Autodesk Fusion 360 part; units mm, degrees
(part 3 of 14)
  arc A556 (6.35, 3.81) -> (6.35, 8.89) centre (6.35, 6.35) ccw
  arc A557 (6.35, 7.62) -> (6.35, 5.08) centre (6.35, 6.35) ccw
  line L1174 (33.239, 57.1172) -> (33.239, 57.7268)
  line L1175 (29.615, 19.102) -> (28.515, 19.102)
  line L1176 (33.872, 57.1172) -> (33.872, 57.7268)
  arc A558 (6.35, 5.08) -> (6.35, 7.62) centre (6.35, 6.35) ccw
  line L1177 (28.94, 19.5132) -> (29.19, 19.5132)
  arc A559 (6.35, 7.62) -> (6.35, 5.08) centre (6.35, 6.35) ccw
  line L1178 (29.615, 20.118) -> (28.515, 20.118)
  line L1179 (82.637, 29.083) -> (83.187, 29.083)
  line L1180 (29.615, 18.502) -> (29.615, 19.102)
  line L1181 (28.557, 18.4972) -> (28.557, 19.1068)
  line L1182 (29.573, 20.1228) -> (29.573, 19.5132)
  line L1183 (34.255, 57.7268) -> (34.255, 57.1172)
  line L1184 (29.573, 19.5132) -> (28.557, 19.5132)
  line L1185 (29.573, 19.1068) -> (29.573, 18.4972)
  line L1186 (83.437, 29.083) -> (83.987, 29.083)
  line L1187 (28.557, 20.1228) -> (29.573, 20.1228)
  arc A560 (34.2967, 57.722) -> (34.2972, 57.722) centre (34.297, 57.722) ccw
  arc A561 (33.1972, 57.122) -> (33.1967, 57.122) centre (33.197, 57.122) ccw
  arc A562 (8.6995, 11.684) -> (4.0005, 11.684) centre (6.35, 11.684) ccw
  line L1188 (33.239, 57.7268) -> (34.255, 57.7268)
  line L1189 (28.515, 18.502) -> (29.615, 18.502)
  line L1190 (28.557, 20.1228) -> (29.573, 20.1228)
  line L1191 (34.422, 57.422) -> (33.872, 57.422)
  line L1192 (29.19, 19.5132) -> (29.19, 20.1228)
  arc A563 (6.35, 6.6992) -> (6.35, 6.0007) centre (6.35, 6.35) ccw
  arc A564 (77.273, 25.0129) -> (77.273, 24.8351) centre (77.273, 24.924) ccw
  arc A565 (4.0005, 11.684) -> (8.6995, 11.684) centre (6.35, 11.684) ccw
  line L1193 (34.255, 57.7268) -> (34.255, 57.1172)
  line L1194 (28.94, 18.4972) -> (29.19, 18.4972)
  line L1195 (33.239, 57.7268) -> (34.255, 57.7268)
  line L1196 (34.255, 57.1172) -> (33.239, 57.1172)
  line L1197 (29.19, 18.4972) -> (29.19, 19.1068)
  line L1198 (28.515, 20.118) -> (28.515, 19.518)
  arc A566 (6.35, 8.89) -> (6.35, 3.81) centre (6.35, 6.35) ccw
  arc A567 (6.35, 5.08) -> (6.35, 7.62) centre (6.35, 6.35) ccw
  line L1199 (28.557, 20.5292) -> (28.557, 21.1388)
  line L1200 (33.872, 57.7268) -> (33.622, 57.7268)
  arc A568 (33.1967, 57.122) -> (33.1972, 57.122) centre (33.197, 57.122) ccw
  line L1201 (29.573, 19.1068) -> (29.573, 18.4972)
  line L1202 (82.637, 29.083) -> (83.187, 29.083)
  line L1203 (28.557, 19.5132) -> (28.557, 20.1228)
  arc A569 (33.1967, 57.722) -> (33.1972, 57.722) centre (33.197, 57.722) ccw
  arc A570 (77.273, 24.8351) -> (77.273, 25.0129) centre (77.273, 24.924) ccw
  line L1204 (29.573, 18.4972) -> (28.557, 18.4972)
  arc A571 (6.35, 3.81) -> (6.35, 8.89) centre (6.35, 6.35) ccw
  line L1205 (34.422, 57.422) -> (33.872, 57.422)
  line L1206 (33.622, 57.1172) -> (33.872, 57.1172)
  line L1207 (33.239, 57.1172) -> (33.239, 57.7268)
  line L1208 (34.255, 57.1172) -> (33.239, 57.1172)
  line L1209 (34.297, 57.722) -> (33.197, 57.722)
  line L1210 (33.197, 57.722) -> (33.197, 57.122)
  arc A572 (33.1972, 57.722) -> (33.1967, 57.722) centre (33.197, 57.722) ccw
  line L1211 (34.297, 57.122) -> (34.297, 57.722)
  line L1212 (28.94, 20.1228) -> (28.94, 19.5132)
  line L1213 (28.515, 19.102) -> (28.515, 18.502)
  arc A573 (6.35, 6.0007) -> (6.35, 6.6992) centre (6.35, 6.35) ccw
  line L1214 (29.615, 19.518) -> (29.615, 20.118)
  line L1215 (7.8317, 13.1657) -> (8.0113, 13.3453)
  line L1216 (28.557, 19.1068) -> (29.573, 19.1068)
  line L1217 (29.573, 20.5292) -> (28.557, 20.5292)
  line L1218 (29.573, 19.5132) -> (28.557, 19.5132)
  arc A574 (6.35, 8.89) -> (6.35, 3.81) centre (6.35, 6.35) ccw
  line L1219 (28.557, 19.5132) -> (28.557, 20.1228)
  arc A575 (6.35, 7.62) -> (6.35, 5.08) centre (6.35, 6.35) ccw
  line L1220 (29.19, 20.1228) -> (28.94, 20.1228)
  line L1221 (28.94, 19.1068) -> (28.94, 18.4972)
  arc A576 (6.35, 7.62) -> (6.35, 5.08) centre (6.35, 6.35) ccw
  line L1222 (29.573, 21.1388) -> (29.573, 20.5292)
  line L1223 (28.515, 21.134) -> (28.515, 20.534)
  arc A577 (78.9432, 34.3535) -> (78.9432, 34.4805) centre (78.9432, 34.417) ccw
  arc A578 (79.5528, 33.3375) -> (79.5528, 33.4645) centre (79.5528, 33.401) ccw
  arc A579 (79.5528, 34.4805) -> (79.5528, 34.3535) centre (79.5528, 34.417) ccw
  line L1224 (78.9432, 33.401) -> (78.9432, 34.417)
  arc A580 (79.5528, 33.4645) -> (79.5528, 33.3375) centre (79.5528, 33.401) ccw
  line L1225 (79.548, 33.359) -> (79.548, 34.459)
  line L1226 (79.5528, 33.401) -> (78.9432, 33.401)
  arc A581 (79.5528, 34.3535) -> (79.5528, 34.4805) centre (79.5528, 34.417) ccw
  line L1227 (79.548, 34.459) -> (78.948, 34.459)
  arc A582 (79.548, 33.3588) -> (79.548, 33.3592) centre (79.548, 33.359) ccw
  arc A583 (79.548, 33.3592) -> (79.548, 33.3588) centre (79.548, 33.359) ccw
  arc A584 (79.548, 34.4592) -> (79.548, 34.4588) centre (79.548, 34.459) ccw
  arc A585 (78.948, 34.4588) -> (78.948, 34.4592) centre (78.948, 34.459) ccw
  line L1228 (78.948, 34.459) -> (78.948, 33.359)
  arc A586 (78.948, 33.3588) -> (78.948, 33.3592) centre (78.948, 33.359) ccw
  arc A587 (79.548, 34.4588) -> (79.548, 34.4592) centre (79.548, 34.459) ccw
  line L1229 (78.948, 33.359) -> (79.548, 33.359)
  line L1230 (78.9432, 34.417) -> (79.5528, 34.417)
  arc A588 (78.9432, 34.4805) -> (78.9432, 34.3535) centre (78.9432, 34.417) ccw
  arc A589 (78.9432, 33.3375) -> (78.9432, 33.4645) centre (78.9432, 33.401) ccw
  arc A590 (78.9432, 33.4645) -> (78.9432, 33.3375) centre (78.9432, 33.401) ccw
  line L1231 (79.5528, 34.417) -> (79.5528, 33.401)
  arc A591 (94.5642, 21.0185) -> (94.5642, 20.8915) centre (94.5642, 20.955) ccw
  arc A592 (94.5642, 20.8915) -> (94.5642, 21.0185) centre (94.5642, 20.955) ccw
  line L1232 (94.5642, 20.572) -> (94.5642, 20.322)
  arc A593 (95.1738, 20.8915) -> (95.1738, 21.0185) centre (95.1738, 20.955) ccw
  line L1233 (94.5642, 20.322) -> (95.1738, 20.322)
  arc A594 (79.5528, 33.3375) -> (79.5528, 33.4645) centre (79.5528, 33.401) ccw
  line L1234 (0, 0) -> (101.6, 0)
  line L1235 (79.5528, 33.784) -> (79.5528, 34.034)
  line L1236 (95.1738, 20.572) -> (94.5642, 20.572)
  line L1237 (78.9432, 33.784) -> (79.5528, 33.784)
  arc A595 (95.1738, 21.0185) -> (95.1738, 20.8915) centre (95.1738, 20.955) ccw
  arc A596 (79.5528, 33.4645) -> (79.5528, 33.3375) centre (79.5528, 33.401) ccw
  line L1238 (0, 63.5) -> (0, 0)
  arc A597 (94.5642, 19.8755) -> (94.5642, 20.0025) centre (94.5642, 19.939) ccw
  line L1239 (101.6, 63.5) -> (0, 63.5)
  line L1240 (95.1738, 20.322) -> (95.1738, 20.572)
  line L1241 (101.6, 0) -> (101.6, 63.5)
  arc A598 (94.5642, 20.0025) -> (94.5642, 19.8755) centre (94.5642, 19.939) ccw
  arc A599 (-0.0635, 0) -> (0.0635, 0) centre (0, 0) ccw
  arc A600 (78.9432, 34.4805) -> (78.9432, 34.3535) centre (78.9432, 34.417) ccw
  arc A601 (78.948, 34.4592) -> (78.948, 34.4588) centre (78.948, 34.459) ccw
  line L1242 (94.869, 20.322) -> (94.869, 19.772)
  line L1243 (34.422, 57.422) -> (33.872, 57.422)
  arc A602 (78.9432, 34.3535) -> (78.9432, 34.4805) centre (78.9432, 34.417) ccw
  line L1244 (28.557, 20.5292) -> (28.557, 21.1388)
  line L1245 (94.869, 20.322) -> (94.869, 19.772)
  line L1246 (79.5528, 34.034) -> (78.9432, 34.034)
  arc A603 (95.1738, 19.8755) -> (95.1738, 20.0025) centre (95.1738, 19.939) ccw
  arc A604 (95.1738, 20.0025) -> (95.1738, 19.8755) centre (95.1738, 19.939) ccw
  arc A605 (78.948, 33.3592) -> (78.948, 33.3588) centre (78.948, 33.359) ccw
  line L1247 (72.39, 34.4805) -> (72.39, 38.481)
  line L1248 (70.612, 21.59) -> (70.612, 32.385)
  line L1249 (79.248, 33.234) -> (79.248, 33.784)
  line L1250 (20.193, 51.054) -> (25.527, 51.054)
  line L1251 (25.527, 49.149) -> (24.384, 49.149)
  line L1252 (7.874, 53.975) -> (7.874, 47.244)
  arc A606 (0.0635, 63.5) -> (-0.0635, 63.5) centre (0, 63.5) ccw
  line L1253 (70.993, 34.29) -> (71.1835, 34.4805)
  line L1254 (24.384, 49.149) -> (22.987, 47.752)
  line L1255 (71.1581, 19.5148) -> (70.9003, 19.7726)
  line L1256 (22.987, 47.752) -> (20.193, 47.752)
  line L1257 (70.9003, 19.7726) -> (68.3387, 19.7726)
  line L1258 (15.494, 35.814) -> (26.035, 35.814)
  line L1259 (86.3702, 32.9565) -> (86.3702, 36.957)
  line L1260 (82.2935, 36.957) -> (82.2935, 32.766)
  line L1261 (85.0265, 32.9565) -> (86.3702, 32.9565)
  line L1262 (82.169, 22.479) -> (84.963, 22.479)
  line L1263 (22.4155, 53.975) -> (7.874, 53.975)
  line L1264 (85.1535, 22.3012) -> (86.233, 22.3012)
  line L1265 (84.836, 32.766) -> (85.0265, 32.9565)
  line L1266 (71.1835, 34.4805) -> (72.39, 34.4805)
  line L1267 (81.407, 21.59) -> (70.612, 21.59)
  line L1268 (26.035, 35.814) -> (28.829, 37.592)
  line L1269 (20.193, 47.752) -> (20.193, 51.054)
  line L1270 (68.3387, 19.7726) -> (68.3387, 15.4991)
  line L1271 (25.527, 51.054) -> (25.527, 49.149)
  line L1272 (37.338, 45.974) -> (37.338, 41.656)
  line L1273 (37.338, 41.656) -> (39.6875, 39.3065)
  line L1274 (28.829, 37.592) -> (28.829, 43.18)
  line L1275 (9.017, 46.101) -> (20.193, 46.101)
  line L1276 (20.193, 46.101) -> (22.4155, 48.3235)
  arc A607 (101.5365, 0) -> (101.6635, 0) centre (101.6, 0) ccw
  arc A608 (101.5365, 63.5) -> (101.6635, 63.5) centre (101.6, 63.5) ccw
  arc A609 (-0.0635, 63.5) -> (0.0635, 63.5) centre (0, 63.5) ccw
  arc A610 (101.6635, 63.5) -> (101.5365, 63.5) centre (101.6, 63.5) ccw
  line L1277 (7.874, 47.244) -> (9.017, 46.101)
  line L1278 (13.335, 43.18) -> (13.335, 37.973)
  line L1279 (28.829, 43.18) -> (13.335, 43.18)
  line L1280 (22.4155, 48.3235) -> (22.4155, 53.975)
  arc A611 (101.6635, 0) -> (101.5365, 0) centre (101.6, 0) ccw
  line L1281 (13.335, 37.973) -> (15.494, 35.814)
  line L1282 (82.2935, 32.766) -> (84.836, 32.766)
  arc A612 (0.0635, 0) -> (-0.0635, 0) centre (0, 0) ccw
  line L1283 (86.3702, 36.957) -> (82.2935, 36.957)
  line L1284 (84.963, 22.479) -> (85.1535, 22.3012)
  line L1285 (86.233, 22.3012) -> (86.233, 18.415)
  line L1286 (86.233, 18.415) -> (82.169, 18.415)
  line L1287 (68.326, 34.29) -> (70.993, 34.29)
  line L1288 (72.39, 38.481) -> (68.326, 38.481)
  line L1289 (68.326, 38.481) -> (68.326, 34.29)
  line L1290 (68.3387, 15.4991) -> (72.3824, 15.4991)
  line L1291 (82.169, 18.415) -> (82.169, 22.479)
  arc A613 (95.169, 20.9968) -> (95.169, 20.9972) centre (95.169, 20.997) ccw
  line L1292 (94.5642, 20.955) -> (95.1738, 20.955)
  line L1293 (39.624, 43.053) -> (39.624, 45.974)
  line L1294 (65.1993, 50.5765) -> (67.752, 50.5765)
  arc A614 (78.9432, 33.3375) -> (78.9432, 33.4645) centre (78.9432, 33.401) ccw
  line L1295 (95.1738, 20.955) -> (95.1738, 19.939)
  line L1296 (78.9432, 34.417) -> (79.5528, 34.417)
  line L1297 (57.8307, 52.8345) -> (57.8307, 49.4081)
  arc A615 (95.169, 19.8968) -> (95.169, 19.8972) centre (95.169, 19.897) ccw
  arc A616 (94.569, 19.8968) -> (94.569, 19.8972) centre (94.569, 19.897) ccw
  arc A617 (95.1738, 19.8755) -> (95.1738, 20.0025) centre (95.1738, 19.939) ccw
  line L1298 (65.1993, 53.3552) -> (65.1993, 50.5765)
  line L1299 (94.869, 21.122) -> (94.869, 20.572)
  line L1300 (94.869, 21.122) -> (94.869, 20.572)
  line L1301 (94.869, 21.122) -> (94.869, 20.572)
  line L1302 (79.5528, 34.417) -> (79.5528, 33.401)
  arc A618 (16.3571, 17.0434) -> (17.054, 17.0434) centre (16.7056, 17.0434) ccw
  line L1303 (78.9432, 33.401) -> (78.9432, 34.417)
  line L1304 (94.869, 20.322) -> (94.869, 19.772)
  line L1305 (61.4655, 52.8345) -> (57.8307, 52.8345)
  line L1306 (95.169, 19.897) -> (95.169, 20.997)
  line L1307 (95.1738, 19.939) -> (94.5642, 19.939)
  line L1308 (94.569, 19.897) -> (95.169, 19.897)
  arc A619 (95.169, 19.8972) -> (95.169, 19.8968) centre (95.169, 19.897) ccw
  line L1309 (61.4655, 51.7639) -> (61.4655, 52.8345)
  line L1310 (41.275, 39.3065) -> (41.275, 41.402)
  line L1311 (60.5015, 51.7639) -> (61.4655, 51.7639)
  line L1312 (57.8307, 49.4081) -> (59.5782, 49.4081)
  arc A620 (95.169, 20.9972) -> (95.169, 20.9968) centre (95.169, 20.997) ccw
  arc A621 (20.798, 16.9748) -> (20.1011, 16.9748) centre (20.4495, 16.9748) ccw
  line L1313 (39.624, 45.974) -> (37.338, 45.974)
  line L1314 (59.5782, 49.4081) -> (59.5782, 50.8406)
  line L1315 (95.1738, 20.955) -> (95.1738, 19.939)
  arc A622 (95.1738, 20.0025) -> (95.1738, 19.8755) centre (95.1738, 19.939) ccw
  arc A623 (95.1738, 20.8915) -> (95.1738, 21.0185) centre (95.1738, 20.955) ccw
  line L1316 (79.5528, 33.401) -> (78.9432, 33.401)
  line L1317 (41.275, 41.402) -> (39.624, 43.053)
  arc A624 (94.569, 19.8972) -> (94.569, 19.8968) centre (94.569, 19.897) ccw
  line L1318 (39.6875, 39.3065) -> (41.275, 39.3065)
  arc A625 (20.1011, 16.9748) -> (20.798, 16.9748) centre (20.4495, 16.9748) ccw
  line L1319 (95.1738, 19.939) -> (94.5642, 19.939)
  line L1320 (94.569, 20.997) -> (94.569, 19.897)
  arc A626 (94.5642, 19.8755) -> (94.5642, 20.0025) centre (94.5642, 19.939) ccw
  arc A627 (78.9432, 33.4645) -> (78.9432, 33.3375) centre (78.9432, 33.401) ccw
  arc A628 (94.5642, 20.0025) -> (94.5642, 19.8755) centre (94.5642, 19.939) ccw
  line L1321 (59.5782, 50.8406) -> (60.5015, 51.7639)
  line L1322 (81.407, 32.385) -> (81.407, 21.59)
  arc A629 (94.5642, 21.0185) -> (94.5642, 20.8915) centre (94.5642, 20.955) ccw
  arc A630 (94.5642, 20.8915) -> (94.5642, 21.0185) centre (94.5642, 20.955) ccw
  line L1323 (67.752, 53.3552) -> (65.1993, 53.3552)
  arc A631 (17.054, 17.0434) -> (16.3571, 17.0434) centre (16.7056, 17.0434) ccw
  line L1324 (70.612, 32.385) -> (81.407, 32.385)
  arc A632 (94.569, 20.9968) -> (94.569, 20.9972) centre (94.569, 20.997) ccw
  line L1325 (67.752, 50.5765) -> (67.752, 53.3552)
  line L1326 (95.169, 20.997) -> (94.569, 20.997)
  line L1327 (94.5642, 20.955) -> (95.1738, 20.955)
  arc A633 (94.569, 20.9972) -> (94.569, 20.9968) centre (94.569, 20.997) ccw
  arc A634 (95.1738, 21.0185) -> (95.1738, 20.8915) centre (95.1738, 20.955) ccw
  line L1328 (94.5642, 19.939) -> (94.5642, 20.955)
  line L1329 (94.5642, 19.939) -> (94.5642, 20.955)
  line L1330 (93.98, 54.356) -> (95.758, 54.356)
  line L1331 (17.272, 13.081) -> (27.559, 13.081)
  line L1332 (93.853, 24.638) -> (93.853, 23.368)
  line L1333 (15.907, 41.0492) -> (15.907, 44.4528)
  line L1334 (14.129, 41.0492) -> (15.907, 41.0492)
  arc A635 (15.918, 41.0512) -> (15.918, 41.0507) centre (15.918, 41.051) ccw
  arc A636 (15.918, 44.4508) -> (15.918, 44.4513) centre (15.918, 44.451) ccw
  arc A637 (14.118, 44.4508) -> (14.118, 44.4513) centre (14.118, 44.451) ccw
  line L1335 (91.44, 54.61) -> (93.853, 54.61)
  line L1336 (79.248, 33.234) -> (79.248, 33.784)
  line L1337 (78.9432, 34.034) -> (78.9432, 33.784)
  arc A638 (15.907, 41.1127) -> (15.907, 40.9857) centre (15.907, 41.0492) ccw
  line L1338 (95.758, 51.816) -> (93.98, 51.816)
  line L1339 (91.44, 24.638) -> (93.853, 24.638)
  line L1340 (93.98, 21.844) -> (93.98, 24.384)
  line L1341 (95.758, 21.844) -> (93.98, 21.844)
  line L1342 (93.98, 40.894) -> (95.758, 40.894)
  line L1343 (91.313, 39.37) -> (93.726, 39.37)
  line L1344 (27.559, 23.241) -> (17.272, 23.241)
  line L1345 (62.103, 41.402) -> (62.103, 17.526)
  line L1346 (93.853, 53.34) -> (91.44, 53.34)
  line L1347 (93.726, 38.1) -> (91.313, 38.1)
  line L1348 (79.248, 33.234) -> (79.248, 33.784)
  line L1349 (62.103, 17.526) -> (38.354, 17.526)
  line L1350 (93.726, 39.37) -> (93.726, 38.1)
  line L1351 (38.354, 17.526) -> (38.354, 41.402)
  line L1352 (72.3824, 15.4991) -> (72.3824, 19.5148)
  line L1353 (94.107, 6.858) -> (94.107, 9.398)
  line L1354 (72.3824, 19.5148) -> (71.1581, 19.5148)
  line L1355 (93.98, 51.816) -> (93.98, 54.356)
  line L1356 (94.107, 9.525) -> (91.567, 9.525)
  arc A639 (79.5528, 34.3535) -> (79.5528, 34.4805) centre (79.5528, 34.417) ccw
  arc A640 (15.907, 44.3893) -> (15.907, 44.5163) centre (15.907, 44.4528) ccw
  line L1357 (91.44, 23.368) -> (91.44, 24.638)
  line L1358 (95.885, 9.398) -> (95.885, 6.858)
  line L1359 (93.98, 24.384) -> (95.758, 24.384)
  line L1360 (95.758, 24.384) -> (95.758, 21.844)
  line L1361 (93.98, 38.354) -> (93.98, 40.894)
  line L1362 (91.313, 38.1) -> (91.313, 39.37)
  line L1363 (95.758, 54.356) -> (95.758, 51.816)
  line L1364 (95.885, 6.858) -> (94.107, 6.858)
  line L1365 (17.272, 23.241) -> (17.272, 13.081)
  line L1366 (91.44, 53.34) -> (91.44, 54.61)
  line L1367 (27.559, 13.081) -> (27.559, 23.241)
  line L1368 (95.758, 40.894) -> (95.758, 38.354)
  line L1369 (38.354, 41.402) -> (62.103, 41.402)
  line L1370 (91.567, 10.795) -> (94.107, 10.795)
  line L1371 (93.853, 23.368) -> (91.44, 23.368)
  line L1372 (93.853, 54.61) -> (93.853, 53.34)
  line L1373 (94.107, 10.795) -> (94.107, 9.525)
  line L1374 (91.567, 9.525) -> (91.567, 10.795)
  arc A641 (79.5528, 34.4805) -> (79.5528, 34.3535) centre (79.5528, 34.417) ccw
  line L1375 (14.129, 41.0492) -> (15.907, 41.0492)
  arc A642 (14.129, 44.3893) -> (14.129, 44.5163) centre (14.129, 44.4528) ccw
  line L1376 (14.129, 44.4528) -> (14.129, 41.0492)
  line L1377 (15.918, 41.051) -> (15.918, 44.451)
  line L1378 (14.129, 44.4528) -> (14.129, 41.0492)
  line L1379 (15.907, 44.4528) -> (14.129, 44.4528)
  line L1380 (95.758, 38.354) -> (93.98, 38.354)
  line L1381 (94.107, 9.398) -> (95.885, 9.398)
  arc A643 (23.992, 42.9753) -> (23.992, 42.9748) centre (23.992, 42.975) ccw
  arc A644 (14.129, 44.5163) -> (14.129, 44.3893) centre (14.129, 44.4528) ccw
  arc A645 (14.118, 44.4513) -> (14.118, 44.4508) centre (14.118, 44.451) ccw
  arc A646 (14.129, 40.9857) -> (14.129, 41.1127) centre (14.129, 41.0492) ccw
  line L1382 (14.168, 41.351) -> (15.868, 41.351)
  arc A647 (25.792, 42.9753) -> (25.792, 42.9748) centre (25.792, 42.975) ccw
  line L1383 (15.918, 44.451) -> (14.118, 44.451)
  arc A648 (15.907, 40.9857) -> (15.907, 41.1127) centre (15.907, 41.0492) ccw
  line L1384 (14.118, 41.051) -> (15.918, 41.051)
  arc A649 (25.792, 39.5752) -> (25.792, 39.5747) centre (25.792, 39.575) ccw
  line L1385 (23.992, 42.975) -> (23.992, 39.575)
  arc A650 (15.907, 41.1127) -> (15.907, 40.9857) centre (15.907, 41.0492) ccw
  line L1386 (14.168, 44.151) -> (15.868, 44.151)
  line L1387 (24.003, 39.5732) -> (25.781, 39.5732)
  line L1388 (25.781, 39.5732) -> (25.781, 42.9768)
  arc A651 (23.992, 39.5747) -> (23.992, 39.5752) centre (23.992, 39.575) ccw
  line L1389 (25.781, 42.9768) -> (24.003, 42.9768)
  arc A652 (25.792, 42.9748) -> (25.792, 42.9753) centre (25.792, 42.975) ccw
  arc A653 (24.003, 39.5097) -> (24.003, 39.6367) centre (24.003, 39.5732) ccw
  arc A654 (25.781, 39.6367) -> (25.781, 39.5097) centre (25.781, 39.5732) ccw
  arc A655 (24.003, 39.6367) -> (24.003, 39.5097) centre (24.003, 39.5732) ccw
  arc A656 (25.781, 43.0403) -> (25.781, 42.9133) centre (25.781, 42.9768) ccw
  arc A657 (24.003, 42.9133) -> (24.003, 43.0403) centre (24.003, 42.9768) ccw
  arc A658 (24.003, 43.0403) -> (24.003, 42.9133) centre (24.003, 42.9768) ccw
  arc A659 (14.129, 44.5163) -> (14.129, 44.3893) centre (14.129, 44.4528) ccw
  arc A660 (25.792, 39.5747) -> (25.792, 39.5752) centre (25.792, 39.575) ccw
  arc A661 (23.992, 42.9748) -> (23.992, 42.9753) centre (23.992, 42.975) ccw
  line L1390 (24.003, 42.9768) -> (24.003, 39.5732)
  arc A662 (14.129, 41.1127) -> (14.129, 40.9857) centre (14.129, 41.0492) ccw
  arc A663 (14.129, 44.3893) -> (14.129, 44.5163) centre (14.129, 44.4528) ccw
  arc A664 (15.907, 44.3893) -> (15.907, 44.5163) centre (15.907, 44.4528) ccw
  arc A665 (14.129, 44.5163) -> (14.129, 44.3893) centre (14.129, 44.4528) ccw
  arc A666 (14.129, 44.5163) -> (14.129, 44.3893) centre (14.129, 44.4528) ccw
  line L1391 (14.168, 41.351) -> (15.868, 41.351)
  line L1392 (14.118, 44.451) -> (14.118, 41.051)
  arc A667 (15.918, 41.0507) -> (15.918, 41.0512) centre (15.918, 41.051) ccw
  arc A668 (15.907, 44.5163) -> (15.907, 44.3893) centre (15.907, 44.4528) ccw
  arc A669 (14.118, 41.0507) -> (14.118, 41.0512) centre (14.118, 41.051) ccw
  arc A670 (14.129, 41.1127) -> (14.129, 40.9857) centre (14.129, 41.0492) ccw
  line L1393 (25.792, 39.575) -> (25.792, 42.975)
  line L1394 (14.168, 44.151) -> (15.868, 44.151)
  arc A671 (14.129, 44.3893) -> (14.129, 44.5163) centre (14.129, 44.4528) ccw
  arc A672 (23.992, 39.5752) -> (23.992, 39.5747) centre (23.992, 39.575) ccw
  line L1395 (15.907, 41.0492) -> (15.907, 44.4528)
  line L1396 (15.907, 44.4528) -> (14.129, 44.4528)
  arc A673 (15.907, 44.5163) -> (15.907, 44.3893) centre (15.907, 44.4528) ccw
  arc A674 (14.129, 44.3893) -> (14.129, 44.5163) centre (14.129, 44.4528) ccw
  line L1397 (79.248, 34.034) -> (79.248, 34.584)
  arc A675 (15.918, 44.4513) -> (15.918, 44.4508) centre (15.918, 44.451) ccw
  arc A676 (14.129, 40.9857) -> (14.129, 41.1127) centre (14.129, 41.0492) ccw
  line L1398 (79.248, 34.034) -> (79.248, 34.584)
  arc A677 (14.118, 41.0512) -> (14.118, 41.0507) centre (14.118, 41.051) ccw
  arc A678 (15.907, 40.9857) -> (15.907, 41.1127) centre (15.907, 41.0492) ccw
  line L1399 (79.248, 34.034) -> (79.248, 34.584)
  line L1400 (14.168, 44.151) -> (15.868, 44.151)
  line L1401 (23.992, 39.575) -> (25.792, 39.575)
  line L1402 (25.792, 42.975) -> (23.992, 42.975)
  line L1403 (14.168, 41.351) -> (15.868, 41.351)
  line L1404 (24.042, 42.675) -> (25.742, 42.675)
  arc A679 (10.922, 53.4543) -> (10.922, 53.5813) centre (10.922, 53.5178) ccw
  line L1405 (9.144, 53.5178) -> (9.144, 50.1142)
  line L1406 (9.133, 50.116) -> (10.933, 50.116)
  arc A680 (9.144, 53.5813) -> (9.144, 53.4543) centre (9.144, 53.5178) ccw
  line L1407 (24.042, 39.875) -> (25.742, 39.875)
  arc A681 (9.144, 50.1777) -> (9.144, 50.0507) centre (9.144, 50.1142) ccw
  arc A682 (24.003, 43.0403) -> (24.003, 42.9133) centre (24.003, 42.9768) ccw
  arc A683 (9.144, 53.4543) -> (9.144, 53.5813) centre (9.144, 53.5178) ccw
  line L1408 (24.003, 42.9768) -> (24.003, 39.5732)
  line L1409 (25.781, 42.9768) -> (24.003, 42.9768)
  line L1410 (10.922, 50.1142) -> (10.922, 53.5178)
  arc A684 (10.922, 53.4543) -> (10.922, 53.5813) centre (10.922, 53.5178) ccw
  arc A685 (10.922, 50.0507) -> (10.922, 50.1777) centre (10.922, 50.1142) ccw
  arc A686 (10.933, 50.1157) -> (10.933, 50.1162) centre (10.933, 50.116) ccw
  line L1411 (9.133, 53.516) -> (9.133, 50.116)
  arc A687 (9.133, 53.5163) -> (9.133, 53.5158) centre (9.133, 53.516) ccw
  arc A688 (9.133, 53.5158) -> (9.133, 53.5163) centre (9.133, 53.516) ccw
  arc A689 (24.003, 42.9133) -> (24.003, 43.0403) centre (24.003, 42.9768) ccw
  arc A690 (25.781, 39.5097) -> (25.781, 39.6367) centre (25.781, 39.5732) ccw
  arc A691 (9.144, 53.5813) -> (9.144, 53.4543) centre (9.144, 53.5178) ccw
  arc A692 (24.003, 42.9133) -> (24.003, 43.0403) centre (24.003, 42.9768) ccw
  arc A693 (24.003, 43.0403) -> (24.003, 42.9133) centre (24.003, 42.9768) ccw
  arc A694 (10.933, 50.1162) -> (10.933, 50.1157) centre (10.933, 50.116) ccw
  arc A695 (9.144, 53.4543) -> (9.144, 53.5813) centre (9.144, 53.5178) ccw
  arc A696 (9.144, 50.1777) -> (9.144, 50.0507) centre (9.144, 50.1142) ccw
  line L1412 (10.922, 53.5178) -> (9.144, 53.5178)
  arc A697 (9.144, 50.0507) -> (9.144, 50.1777) centre (9.144, 50.1142) ccw
  line L1413 (24.042, 42.675) -> (25.742, 42.675)
  arc A698 (10.922, 50.1777) -> (10.922, 50.0507) centre (10.922, 50.1142) ccw
  arc A699 (9.144, 53.5813) -> (9.144, 53.4543) centre (9.144, 53.5178) ccw
  arc A700 (24.003, 43.0403) -> (24.003, 42.9133) centre (24.003, 42.9768) ccw
  line L1414 (10.933, 50.116) -> (10.933, 53.516)
  arc A701 (10.922, 50.0507) -> (10.922, 50.1777) centre (10.922, 50.1142) ccw
  arc A702 (10.922, 53.5813) -> (10.922, 53.4543) centre (10.922, 53.5178) ccw
  arc A703 (10.933, 53.5163) -> (10.933, 53.5158) centre (10.933, 53.516) ccw
  arc A704 (10.922, 50.1777) -> (10.922, 50.0507) centre (10.922, 50.1142) ccw
  line L1415 (24.003, 39.5732) -> (25.781, 39.5732)
  arc A705 (10.933, 53.5158) -> (10.933, 53.5163) centre (10.933, 53.516) ccw
  arc A706 (9.133, 50.1162) -> (9.133, 50.1157) centre (9.133, 50.116) ccw
  arc A707 (9.144, 53.4543) -> (9.144, 53.5813) centre (9.144, 53.5178) ccw
  arc A708 (25.781, 42.9133) -> (25.781, 43.0403) centre (25.781, 42.9768) ccw
  arc A709 (25.781, 39.6367) -> (25.781, 39.5097) centre (25.781, 39.5732) ccw
  arc A710 (24.003, 39.6367) -> (24.003, 39.5097) centre (24.003, 39.5732) ccw
  line L1416 (25.781, 39.5732) -> (25.781, 42.9768)
  line L1417 (24.042, 39.875) -> (25.742, 39.875)
  line L1418 (9.144, 50.1142) -> (10.922, 50.1142)
  line L1419 (9.144, 53.5178) -> (9.144, 50.1142)
  arc A711 (25.781, 39.5097) -> (25.781, 39.6367) centre (25.781, 39.5732) ccw
  arc A712 (9.144, 50.0507) -> (9.144, 50.1777) centre (9.144, 50.1142) ccw
  line L1420 (24.042, 42.675) -> (25.742, 42.675)
  arc A713 (24.003, 39.5097) -> (24.003, 39.6367) centre (24.003, 39.5732) ccw
  arc A714 (24.003, 42.9133) -> (24.003, 43.0403) centre (24.003, 42.9768) ccw
  line L1421 (10.933, 53.516) -> (9.133, 53.516)
  arc A715 (25.781, 43.0403) -> (25.781, 42.9133) centre (25.781, 42.9768) ccw
  line L1422 (10.922, 53.5178) -> (9.144, 53.5178)
  arc A716 (25.781, 42.9133) -> (25.781, 43.0403) centre (25.781, 42.9768) ccw
  line L1423 (24.042, 39.875) -> (25.742, 39.875)
  line L1424 (80.564, 33.359) -> (80.564, 34.459)
  arc A717 (79.964, 34.4592) -> (79.964, 34.4588) centre (79.964, 34.459) ccw
  line L1425 (79.9592, 34.417) -> (80.5688, 34.417)
  line L1426 (79.9592, 33.401) -> (79.9592, 34.417)
  line L1427 (80.5688, 34.417) -> (80.5688, 33.401)
  line L1428 (80.264, 34.034) -> (80.264, 34.584)
  arc A718 (80.5688, 34.3535) -> (80.5688, 34.4805) centre (80.5688, 34.417) ccw
  line L1429 (20.18, 51.238) -> (21.98, 51.238)
  line L1430 (79.9592, 33.401) -> (79.9592, 34.417)
  line L1431 (80.264, 33.234) -> (80.264, 33.784)
  line L1432 (10.922, 50.1142) -> (10.922, 53.5178)
  arc A719 (79.9592, 33.4645) -> (79.9592, 33.3375) centre (79.9592, 33.401) ccw
  arc A720 (9.144, 53.5813) -> (9.144, 53.4543) centre (9.144, 53.5178) ccw
  arc A721 (79.964, 34.4588) -> (79.964, 34.4592) centre (79.964, 34.459) ccw
  line L1433 (80.264, 33.234) -> (80.264, 33.784)
  line L1434 (9.183, 50.416) -> (10.883, 50.416)
  line L1435 (80.5688, 33.401) -> (79.9592, 33.401)
  arc A722 (79.9592, 33.4645) -> (79.9592, 33.3375) centre (79.9592, 33.401) ccw
  line L1436 (20.18, 54.638) -> (20.18, 51.238)
  line L1437 (79.9592, 34.417) -> (80.5688, 34.417)
  line L1438 (9.183, 50.416) -> (10.883, 50.416)
  line L1439 (80.5688, 33.784) -> (80.5688, 34.034)
  arc A723 (79.9592, 34.4805) -> (79.9592, 34.3535) centre (79.9592, 34.417) ccw
  arc A724 (79.9592, 33.3375) -> (79.9592, 33.4645) centre (79.9592, 33.401) ccw
  arc A725 (80.564, 34.4588) -> (80.564, 34.4592) centre (80.564, 34.459) ccw
  arc A726 (79.9592, 34.3535) -> (79.9592, 34.4805) centre (79.9592, 34.417) ccw
  arc A727 (80.5688, 33.3375) -> (80.5688, 33.4645) centre (80.5688, 33.401) ccw
  line L1440 (80.264, 34.034) -> (80.264, 34.584)
  arc A728 (10.922, 53.5813) -> (10.922, 53.4543) centre (10.922, 53.5178) ccw
  line L1441 (9.183, 53.216) -> (10.883, 53.216)
  line L1442 (80.5688, 34.417) -> (80.5688, 33.401)
  arc A729 (9.133, 50.1157) -> (9.133, 50.1162) centre (9.133, 50.116) ccw
  line L1443 (80.5688, 33.401) -> (79.9592, 33.401)
  arc A730 (9.144, 53.4543) -> (9.144, 53.5813) centre (9.144, 53.5178) ccw
  arc A731 (79.964, 33.3588) -> (79.964, 33.3592) centre (79.964, 33.359) ccw
  arc A732 (80.5688, 33.4645) -> (80.5688, 33.3375) centre (80.5688, 33.401) ccw
  arc A733 (80.5688, 33.3375) -> (80.5688, 33.4645) centre (80.5688, 33.401) ccw
  arc A734 (79.964, 33.3592) -> (79.964, 33.3588) centre (79.964, 33.359) ccw
  arc A735 (79.9592, 33.3375) -> (79.9592, 33.4645) centre (79.9592, 33.401) ccw
  arc A736 (79.9592, 34.3535) -> (79.9592, 34.4805) centre (79.9592, 34.417) ccw
  line L1444 (9.144, 50.1142) -> (10.922, 50.1142)
  line L1445 (80.564, 34.459) -> (79.964, 34.459)
  line L1446 (79.9592, 33.784) -> (80.5688, 33.784)
  line L1447 (79.964, 33.359) -> (80.564, 33.359)
  arc A737 (80.5688, 33.4645) -> (80.5688, 33.3375) centre (80.5688, 33.401) ccw
  line L1448 (9.183, 50.416) -> (10.883, 50.416)
  line L1449 (9.183, 53.216) -> (10.883, 53.216)
  arc A738 (80.5688, 34.4805) -> (80.5688, 34.3535) centre (80.5688, 34.417) ccw
  line L1450 (80.5688, 34.034) -> (79.9592, 34.034)
  line L1451 (79.964, 34.459) -> (79.964, 33.359)
  arc A739 (80.564, 33.3588) -> (80.564, 33.3592) centre (80.564, 33.359) ccw
  arc A740 (80.564, 33.3592) -> (80.564, 33.3588) centre (80.564, 33.359) ccw
  line L1452 (9.183, 53.216) -> (10.883, 53.216)
  arc A741 (80.564, 34.4592) -> (80.564, 34.4588) centre (80.564, 34.459) ccw
  arc A742 (79.9592, 34.4805) -> (79.9592, 34.3535) centre (79.9592, 34.417) ccw
  line L1453 (80.264, 33.234) -> (80.264, 33.784)
  line L1454 (80.264, 34.034) -> (80.264, 34.584)
  arc A743 (80.5688, 34.4805) -> (80.5688, 34.3535) centre (80.5688, 34.417) ccw
  line L1455 (79.9592, 34.034) -> (79.9592, 33.784)
  arc A744 (80.5688, 34.3535) -> (80.5688, 34.4805) centre (80.5688, 34.417) ccw
  arc A745 (21.969, 51.2997) -> (21.969, 51.1727) centre (21.969, 51.2362) ccw
  arc A746 (3.048, 52.3875) -> (3.048, 52.5145) centre (3.048, 52.451) ccw
  line L1456 (21.969, 54.6398) -> (20.191, 54.6398)
  line L1457 (3.048, 44.831) -> (7.62, 44.831)
  line L1458 (3.048, 52.451) -> (3.048, 44.831)
  arc A747 (3.048, 52.5145) -> (3.048, 52.3875) centre (3.048, 52.451) ccw
  arc A748 (3.048, 52.3875) -> (3.048, 52.5145) centre (3.048, 52.451) ccw
  arc A749 (20.191, 54.5763) -> (20.191, 54.7033) centre (20.191, 54.6398) ccw
  line L1459 (7.5946, 51.8668) -> (7.5946, 52.0446)
  line L1460 (21.969, 54.6398) -> (20.191, 54.6398)
  line L1461 (20.23, 54.338) -> (21.93, 54.338)
  line L1462 (20.191, 51.2362) -> (21.969, 51.2362)
  line L1463 (3.1242, 52.0446) -> (3.1242, 52.2478)
  line L1464 (20.23, 54.338) -> (21.93, 54.338)
  arc A750 (7.5946, 51.9303) -> (7.5946, 51.8033) centre (7.5946, 51.8668) ccw
  arc A751 (3.048, 44.8945) -> (3.048, 44.7675) centre (3.048, 44.831) ccw
  line L1465 (7.62, 44.831) -> (7.62, 52.451)
  arc A752 (3.1242, 52.1081) -> (3.1242, 51.9811) centre (3.1242, 52.0446) ccw
  arc A753 (7.5946, 52.1081) -> (7.5946, 51.9811) centre (7.5946, 52.0446) ccw
  arc A754 (20.191, 54.5763) -> (20.191, 54.7033) centre (20.191, 54.6398) ccw
  arc A755 (20.191, 54.7033) -> (20.191, 54.5763) centre (20.191, 54.6398) ccw
  arc A756 (21.969, 51.2997) -> (21.969, 51.1727) centre (21.969, 51.2362) ccw
  arc A757 (20.191, 51.2997) -> (20.191, 51.1727) centre (20.191, 51.2362) ccw
  line L1466 (21.98, 51.238) -> (21.98, 54.638)
  arc A758 (20.191, 51.1727) -> (20.191, 51.2997) centre (20.191, 51.2362) ccw
  line L1467 (20.191, 54.6398) -> (20.191, 51.2362)
  line L1468 (3.0988, 51.8668) -> (7.5946, 51.8668)
  line L1469 (21.969, 51.2362) -> (21.969, 54.6398)
  line L1470 (20.191, 54.6398) -> (20.191, 51.2362)
  arc A759 (20.191, 54.7033) -> (20.191, 54.5763) centre (20.191, 54.6398) ccw
  line L1471 (20.23, 54.338) -> (21.93, 54.338)
  line L1472 (3.1242, 52.2478) -> (7.5946, 52.2478)
  arc A760 (21.969, 54.5763) -> (21.969, 54.7033) centre (21.969, 54.6398) ccw
  arc A761 (3.1242, 52.3113) -> (3.1242, 52.1843) centre (3.1242, 52.2478) ccw
  arc A762 (3.048, 52.5145) -> (3.048, 52.3875) centre (3.048, 52.451) ccw
  arc A763 (7.62, 44.8945) -> (7.62, 44.7675) centre (7.62, 44.831) ccw
  line L1473 (20.23, 51.538) -> (21.93, 51.538)
  arc A764 (21.969, 51.1727) -> (21.969, 51.2997) centre (21.969, 51.2362) ccw
  arc A765 (21.98, 54.6378) -> (21.98, 54.6382) centre (21.98, 54.638) ccw
  arc A766 (21.98, 51.2377) -> (21.98, 51.2382) centre (21.98, 51.238) ccw
  line L1474 (20.23, 51.538) -> (21.93, 51.538)
  arc A767 (20.191, 51.2997) -> (20.191, 51.1727) centre (20.191, 51.2362) ccw
  arc A768 (20.18, 51.2377) -> (20.18, 51.2382) centre (20.18, 51.238) ccw
  arc A769 (20.191, 54.5763) -> (20.191, 54.7033) centre (20.191, 54.6398) ccw
  arc A770 (20.18, 51.2382) -> (20.18, 51.2377) centre (20.18, 51.238) ccw
  line L1475 (21.969, 51.2362) -> (21.969, 54.6398)
  arc A771 (20.191, 54.7033) -> (20.191, 54.5763) centre (20.191, 54.6398) ccw
  arc A772 (20.191, 51.1727) -> (20.191, 51.2997) centre (20.191, 51.2362) ccw
  line L1476 (21.98, 54.638) -> (20.18, 54.638)
  arc A773 (21.969, 54.7033) -> (21.969, 54.5763) centre (21.969, 54.6398) ccw
  line L1477 (20.191, 51.2362) -> (21.969, 51.2362)
  arc A774 (21.969, 54.5763) -> (21.969, 54.7033) centre (21.969, 54.6398) ccw
  arc A775 (20.191, 54.5763) -> (20.191, 54.7033) centre (20.191, 54.6398) ccw
  arc A776 (21.98, 51.2382) -> (21.98, 51.2377) centre (21.98, 51.238) ccw
  arc A777 (7.5946, 51.8033) -> (7.5946, 51.9303) centre (7.5946, 51.8668) ccw
  arc A778 (20.191, 54.7033) -> (20.191, 54.5763) centre (20.191, 54.6398) ccw
  arc A779 (20.18, 54.6378) -> (20.18, 54.6382) centre (20.18, 54.638) ccw
  arc A780 (21.98, 54.6382) -> (21.98, 54.6378) centre (21.98, 54.638) ccw
  arc A781 (20.18, 54.6382) -> (20.18, 54.6378) centre (20.18, 54.638) ccw
  arc A782 (21.969, 54.7033) -> (21.969, 54.5763) centre (21.969, 54.6398) ccw
  arc A783 (21.969, 51.1727) -> (21.969, 51.2997) centre (21.969, 51.2362) ccw
  arc A784 (7.1374, 53.4289) -> (7.1374, 53.3019) centre (7.1374, 53.3654) ccw
  line L1478 (79.4512, 47.115) -> (79.4512, 46.865)
  arc A785 (80.0608, 46.5455) -> (80.0608, 46.4185) centre (80.0608, 46.482) ccw
  arc A786 (80.0608, 46.5455) -> (80.0608, 46.4185) centre (80.0608, 46.482) ccw
  arc A787 (80.0608, 47.4345) -> (80.0608, 47.5615) centre (80.0608, 47.498) ccw
  arc A788 (3.048, 52.5145) -> (3.048, 52.3875) centre (3.048, 52.451) ccw
  line L1479 (3.048, 44.831) -> (7.62, 44.831)
  arc A789 (79.4512, 46.4185) -> (79.4512, 46.5455) centre (79.4512, 46.482) ccw
  arc A790 (79.4512, 47.5615) -> (79.4512, 47.4345) centre (79.4512, 47.498) ccw
  arc A791 (3.1242, 51.9811) -> (3.1242, 52.1081) centre (3.1242, 52.0446) ccw
  arc A792 (3.048, 44.7675) -> (3.048, 44.8945) centre (3.048, 44.831) ccw
  arc A793 (7.9502, 53.3019) -> (7.9502, 53.4289) centre (7.9502, 53.3654) ccw
  line L1480 (80.056, 46.44) -> (80.056, 47.54)
  arc A794 (80.056, 47.5398) -> (80.056, 47.5402) centre (80.056, 47.54) ccw
  arc A795 (7.5946, 51.9811) -> (7.5946, 52.1081) centre (7.5946, 52.0446) ccw
  arc A796 (3.048, 44.7675) -> (3.048, 44.8945) centre (3.048, 44.831) ccw
  line L1481 (20.23, 51.538) -> (21.93, 51.538)
  arc A797 (7.62, 52.5145) -> (7.62, 52.3875) centre (7.62, 52.451) ccw
  line L1482 (7.5946, 52.0446) -> (3.1242, 52.0446)
  arc A798 (7.5438, 53.8099) -> (7.5438, 53.6829) centre (7.5438, 53.7464) ccw
  arc A799 (7.62, 44.7675) -> (7.62, 44.8945) centre (7.62, 44.831) ccw
  arc A800 (3.0988, 51.9303) -> (3.0988, 51.8033) centre (3.0988, 51.8668) ccw
  line L1483 (4.0386, 51.689) -> (6.6294, 51.689)
  arc A801 (7.1374, 53.3019) -> (7.1374, 53.4289) centre (7.1374, 53.3654) ccw
  line L1484 (80.0608, 47.498) -> (80.0608, 46.482)
  line L1485 (80.0608, 47.498) -> (80.0608, 46.482)
  arc A802 (80.0608, 47.5615) -> (80.0608, 47.4345) centre (80.0608, 47.498) ccw
  line L1486 (4.0386, 45.593) -> (6.6294, 45.593)
  line L1487 (80.0608, 47.115) -> (79.4512, 47.115)
  line L1488 (4.0386, 51.689) -> (6.6294, 51.689)
  arc A803 (79.4512, 46.5455) -> (79.4512, 46.4185) centre (79.4512, 46.482) ccw
  line L1489 (80.056, 47.54) -> (79.456, 47.54)
  arc A804 (7.9502, 53.4289) -> (7.9502, 53.3019) centre (7.9502, 53.3654) ccw
  arc A805 (7.62, 52.3875) -> (7.62, 52.5145) centre (7.62, 52.451) ccw
  line L1490 (79.4512, 46.865) -> (80.0608, 46.865)
  line L1491 (7.9502, 53.3654) -> (7.1374, 53.3654)
  line L1492 (79.456, 47.54) -> (79.456, 46.44)
  line L1493 (7.62, 52.451) -> (3.048, 52.451)
  arc A806 (3.048, 52.3875) -> (3.048, 52.5145) centre (3.048, 52.451) ccw
  arc A807 (7.5438, 52.8955) -> (7.5438, 53.0225) centre (7.5438, 52.959) ccw
  arc A808 (3.048, 44.8945) -> (3.048, 44.7675) centre (3.048, 44.831) ccw
  line L1494 (7.62, 52.451) -> (3.048, 52.451)
  arc A809 (7.62, 44.7675) -> (7.62, 44.8945) centre (7.62, 44.831) ccw
  arc A810 (7.5438, 53.6829) -> (7.5438, 53.8099) centre (7.5438, 53.7464) ccw
  arc A811 (7.62, 52.5145) -> (7.62, 52.3875) centre (7.62, 52.451) ccw
  arc A812 (7.5438, 53.0225) -> (7.5438, 52.8955) centre (7.5438, 52.959) ccw
  arc A813 (7.62, 44.8945) -> (7.62, 44.7675) centre (7.62, 44.831) ccw
  line L1495 (7.5438, 53.7464) -> (7.5438, 52.959)
  arc A814 (7.5946, 52.1843) -> (7.5946, 52.3113) centre (7.5946, 52.2478) ccw
  arc A815 (80.0608, 46.4185) -> (80.0608, 46.5455) centre (80.0608, 46.482) ccw
  arc A816 (80.056, 46.4402) -> (80.056, 46.4398) centre (80.056, 46.44) ccw
  line L1496 (3.048, 52.451) -> (3.048, 44.831)
  arc A817 (79.456, 47.5402) -> (79.456, 47.5398) centre (79.456, 47.54) ccw
  line L1497 (80.0608, 46.482) -> (79.4512, 46.482)
  line L1498 (7.62, 44.831) -> (7.62, 52.451)
  line L1499 (79.4512, 47.498) -> (80.0608, 47.498)
  arc A818 (3.1242, 52.1843) -> (3.1242, 52.3113) centre (3.1242, 52.2478) ccw
  arc A819 (7.62, 52.3875) -> (7.62, 52.5145) centre (7.62, 52.451) ccw
  arc A820 (3.0988, 51.8033) -> (3.0988, 51.9303) centre (3.0988, 51.8668) ccw
  arc A821 (7.5946, 52.3113) -> (7.5946, 52.1843) centre (7.5946, 52.2478) ccw
  line L1500 (4.0386, 51.689) -> (6.6294, 51.689)
  arc A822 (79.4512, 46.5455) -> (79.4512, 46.4185) centre (79.4512, 46.482) ccw
  line L1501 (79.4512, 47.498) -> (80.0608, 47.498)
  arc A823 (80.0608, 46.4185) -> (80.0608, 46.5455) centre (80.0608, 46.482) ccw
  arc A824 (81.0768, 46.4185) -> (81.0768, 46.5455) centre (81.0768, 46.482) ccw
  arc A825 (80.0608, 47.5615) -> (80.0608, 47.4345) centre (80.0608, 47.498) ccw
  line L1502 (81.072, 47.54) -> (80.472, 47.54)
  arc A826 (80.4672, 46.4185) -> (80.4672, 46.5455) centre (80.4672, 46.482) ccw
  arc A827 (80.4672, 46.5455) -> (80.4672, 46.4185) centre (80.4672, 46.482) ccw
  arc A828 (80.472, 47.5398) -> (80.472, 47.5402) centre (80.472, 47.54) ccw
  arc A829 (81.0768, 46.5455) -> (81.0768, 46.4185) centre (81.0768, 46.482) ccw
  line L1503 (80.0608, 46.865) -> (80.0608, 47.115)
  arc A830 (79.456, 46.4398) -> (79.456, 46.4402) centre (79.456, 46.44) ccw
  line L1504 (79.756, 47.665) -> (79.756, 47.115)
  arc A831 (80.4672, 47.4345) -> (80.4672, 47.5615) centre (80.4672, 47.498) ccw
  line L1505 (79.756, 47.665) -> (79.756, 47.115)
  arc A832 (81.072, 46.4398) -> (81.072, 46.4402) centre (81.072, 46.44) ccw
  arc A833 (79.456, 46.4402) -> (79.456, 46.4398) centre (79.456, 46.44) ccw
  arc A834 (80.4672, 46.5455) -> (80.4672, 46.4185) centre (80.4672, 46.482) ccw
  arc A835 (80.4672, 47.4345) -> (80.4672, 47.5615) centre (80.4672, 47.498) ccw
  arc A836 (80.4672, 47.5615) -> (80.4672, 47.4345) centre (80.4672, 47.498) ccw
  line L1506 (4.0386, 45.593) -> (6.6294, 45.593)
  line L1507 (80.4672, 47.498) -> (81.0768, 47.498)
  arc A837 (79.456, 47.5398) -> (79.456, 47.5402) centre (79.456, 47.54) ccw
  line L1508 (80.772, 47.665) -> (80.772, 47.115)
  line L1509 (81.0768, 46.865) -> (81.0768, 47.115)
  line L1510 (81.072, 46.44) -> (81.072, 47.54)
  arc A838 (81.0768, 47.5615) -> (81.0768, 47.4345) centre (81.0768, 47.498) ccw
  line L1511 (80.4672, 46.482) -> (80.4672, 47.498)
  line L1512 (80.772, 47.665) -> (80.772, 47.115)
  arc A839 (80.472, 46.4402) -> (80.472, 46.4398) centre (80.472, 46.44) ccw
  arc A840 (81.072, 47.5398) -> (81.072, 47.5402) centre (81.072, 47.54) ccw
  arc A841 (80.472, 47.5402) -> (80.472, 47.5398) centre (80.472, 47.54) ccw
  arc A842 (79.4512, 47.4345) -> (79.4512, 47.5615) centre (79.4512, 47.498) ccw
  line L1513 (79.756, 46.865) -> (79.756, 46.315)
  line L1514 (80.472, 47.54) -> (80.472, 46.44)
  line L1515 (79.4512, 46.482) -> (79.4512, 47.498)
  line L1516 (80.0608, 46.482) -> (79.4512, 46.482)
  arc A843 (80.0608, 47.4345) -> (80.0608, 47.5615) centre (80.0608, 47.498) ccw
  arc A844 (79.4512, 46.4185) -> (79.4512, 46.5455) centre (79.4512, 46.482) ccw
  line L1517 (79.456, 46.44) -> (80.056, 46.44)
  arc A845 (81.0768, 47.5615) -> (81.0768, 47.4345) centre (81.0768, 47.498) ccw
  line L1518 (4.0386, 45.593) -> (6.6294, 45.593)
  arc A846 (80.056, 46.4398) -> (80.056, 46.4402) centre (80.056, 46.44) ccw
  arc A847 (80.472, 46.4398) -> (80.472, 46.4402) centre (80.472, 46.44) ccw
  line L1519 (81.0768, 47.498) -> (81.0768, 46.482)
  arc A848 (79.4512, 47.5615) -> (79.4512, 47.4345) centre (79.4512, 47.498) ccw
  arc A849 (79.4512, 47.4345) -> (79.4512, 47.5615) centre (79.4512, 47.498) ccw
  line L1520 (80.4672, 46.482) -> (80.4672, 47.498)
  arc A850 (80.4672, 47.5615) -> (80.4672, 47.4345) centre (80.4672, 47.498) ccw
  line L1521 (79.756, 46.865) -> (79.756, 46.315)
  arc A851 (81.0768, 47.4345) -> (81.0768, 47.5615) centre (81.0768, 47.498) ccw
  line L1522 (80.4672, 47.498) -> (81.0768, 47.498)
  arc A852 (80.056, 47.5402) -> (80.056, 47.5398) centre (80.056, 47.54) ccw
  line L1523 (80.472, 46.44) -> (81.072, 46.44)
  line L1524 (81.0768, 46.482) -> (80.4672, 46.482)
  arc A853 (81.072, 46.4402) -> (81.072, 46.4398) centre (81.072, 46.44) ccw
  arc A854 (81.072, 47.5402) -> (81.072, 47.5398) centre (81.072, 47.54) ccw
  line L1525 (81.0768, 46.482) -> (80.4672, 46.482)
  line L1526 (79.756, 46.865) -> (79.756, 46.315)
  line L1527 (79.4512, 46.482) -> (79.4512, 47.498)
  line L1528 (79.756, 47.665) -> (79.756, 47.115)
  arc A855 (82.088, 47.5402) -> (82.088, 47.5398) centre (82.088, 47.54) ccw
  line L1529 (81.4832, 47.115) -> (81.4832, 46.865)
  line L1530 (82.0928, 47.498) -> (82.0928, 46.482)
  arc A856 (81.488, 47.5402) -> (81.488, 47.5398) centre (81.488, 47.54) ccw
  arc A857 (81.4832, 46.5455) -> (81.4832, 46.4185) centre (81.4832, 46.482) ccw
  arc A858 (81.0768, 46.5455) -> (81.0768, 46.4185) centre (81.0768, 46.482) ccw
  line L1531 (81.788, 47.665) -> (81.788, 47.115)
  arc A859 (83.1088, 46.4185) -> (83.1088, 46.5455) centre (83.1088, 46.482) ccw
  line L1532 (83.1088, 46.482) -> (82.4992, 46.482)
  line L1533 (81.788, 46.865) -> (81.788, 46.315)
  line L1534 (82.0928, 46.865) -> (82.0928, 47.115)
  line L1535 (81.0768, 47.115) -> (80.4672, 47.115)
  arc A860 (82.0928, 47.5615) -> (82.0928, 47.4345) centre (82.0928, 47.498) ccw
  arc A861 (83.104, 47.5402) -> (83.104, 47.5398) centre (83.104, 47.54) ccw
  arc A862 (81.488, 47.5398) -> (81.488, 47.5402) centre (81.488, 47.54) ccw
  arc A863 (81.488, 46.4402) -> (81.488, 46.4398) centre (81.488, 46.44) ccw
  arc A864 (82.0928, 46.4185) -> (82.0928, 46.5455) centre (82.0928, 46.482) ccw
  arc A865 (82.0928, 47.4345) -> (82.0928, 47.5615) centre (82.0928, 47.498) ccw
  arc A866 (81.4832, 46.4185) -> (81.4832, 46.5455) centre (81.4832, 46.482) ccw
  arc A867 (81.4832, 47.4345) -> (81.4832, 47.5615) centre (81.4832, 47.498) ccw
  line L1536 (81.4832, 46.482) -> (81.4832, 47.498)
  arc A868 (81.4832, 47.5615) -> (81.4832, 47.4345) centre (81.4832, 47.498) ccw
  line L1537 (81.4832, 46.865) -> (82.0928, 46.865)
  line L1538 (82.4992, 46.482) -> (82.4992, 47.498)
  line L1539 (81.0768, 47.498) -> (81.0768, 46.482)
  arc A869 (82.088, 46.4402) -> (82.088, 46.4398) centre (82.088, 46.44) ccw
  arc A870 (81.0768, 46.4185) -> (81.0768, 46.5455) centre (81.0768, 46.482) ccw
  arc A871 (81.4832, 46.4185) -> (81.4832, 46.5455) centre (81.4832, 46.482) ccw
  arc A872 (82.504, 47.5402) -> (82.504, 47.5398) centre (82.504, 47.54) ccw
  line L1540 (80.4672, 46.865) -> (81.0768, 46.865)
  line L1541 (80.772, 47.665) -> (80.772, 47.115)
  arc A873 (82.0928, 46.5455) -> (82.0928, 46.4185) centre (82.0928, 46.482) ccw
  line L1542 (81.4832, 47.498) -> (82.0928, 47.498)
  line L1543 (81.488, 47.54) -> (81.488, 46.44)
  line L1544 (82.0928, 47.498) -> (82.0928, 46.482)
  line L1545 (82.0928, 46.482) -> (81.4832, 46.482)
  arc A874 (81.4832, 47.5615) -> (81.4832, 47.4345) centre (81.4832, 47.498) ccw
  line L1546 (81.788, 47.665) -> (81.788, 47.115)
  line L1547 (80.772, 46.865) -> (80.772, 46.315)
  line L1548 (81.488, 46.44) -> (82.088, 46.44)
  arc A875 (81.0768, 47.4345) -> (81.0768, 47.5615) centre (81.0768, 47.498) ccw
  arc A876 (82.0928, 46.5455) -> (82.0928, 46.4185) centre (82.0928, 46.482) ccw
  arc A877 (81.4832, 46.5455) -> (81.4832, 46.4185) centre (81.4832, 46.482) ccw
  line L1549 (82.088, 46.44) -> (82.088, 47.54)
  arc A878 (82.0928, 46.4185) -> (82.0928, 46.5455) centre (82.0928, 46.482) ccw
  line L1550 (81.4832, 46.482) -> (81.4832, 47.498)
  line L1551 (81.788, 47.665) -> (81.788, 47.115)
  arc A879 (82.088, 46.4398) -> (82.088, 46.4402) centre (82.088, 46.44) ccw
  line L1552 (80.4672, 47.115) -> (80.4672, 46.865)
  line L1553 (82.088, 47.54) -> (81.488, 47.54)
  arc A880 (82.088, 47.5398) -> (82.088, 47.5402) centre (82.088, 47.54) ccw
  arc A881 (81.488, 46.4398) -> (81.488, 46.4402) centre (81.488, 46.44) ccw
  arc A882 (82.0928, 47.5615) -> (82.0928, 47.4345) centre (82.0928, 47.498) ccw
  arc A883 (81.4832, 47.4345) -> (81.4832, 47.5615) centre (81.4832, 47.498) ccw
  arc A884 (80.4672, 46.4185) -> (80.4672, 46.5455) centre (80.4672, 46.482) ccw
  line L1554 (82.0928, 47.115) -> (81.4832, 47.115)
  line L1555 (81.4832, 47.498) -> (82.0928, 47.498)
  line L1556 (82.0928, 46.482) -> (81.4832, 46.482)
  line L1557 (80.772, 46.865) -> (80.772, 46.315)
  arc A885 (82.0928, 47.4345) -> (82.0928, 47.5615) centre (82.0928, 47.498) ccw
  line L1558 (80.772, 46.865) -> (80.772, 46.315)
  line L1559 (85.217, 50.9778) -> (85.217, 50.3682)
  line L1560 (84.201, 50.9778) -> (85.217, 50.9778)
  line L1561 (84.159, 50.373) -> (85.259, 50.373)
  arc A886 (85.2592, 50.373) -> (85.2588, 50.373) centre (85.259, 50.373) ccw
  arc A887 (85.1535, 50.9778) -> (85.2805, 50.9778) centre (85.217, 50.9778) ccw
  arc A888 (82.4992, 46.4185) -> (82.4992, 46.5455) centre (82.4992, 46.482) ccw
  line L1562 (83.104, 46.44) -> (83.104, 47.54)
  arc A889 (84.1588, 50.973) -> (84.1592, 50.973) centre (84.159, 50.973) ccw
  line L1563 (82.804, 47.665) -> (82.804, 47.115)
  arc A890 (83.1088, 47.4345) -> (83.1088, 47.5615) centre (83.1088, 47.498) ccw
  line L1564 (82.4992, 47.498) -> (83.1088, 47.498)
  line L1565 (81.788, 46.865) -> (81.788, 46.315)
  arc A891 (85.2588, 50.973) -> (85.2592, 50.973) centre (85.259, 50.973) ccw
  line L1566 (85.259, 50.973) -> (84.159, 50.973)
  arc A892 (83.104, 46.4398) -> (83.104, 46.4402) centre (83.104, 46.44) ccw
  line L1567 (83.1088, 47.498) -> (83.1088, 46.482)
  line L1568 (81.788, 46.865) -> (81.788, 46.315)
  arc A893 (82.4992, 47.4345) -> (82.4992, 47.5615) centre (82.4992, 47.498) ccw
  arc A894 (83.1088, 46.5455) -> (83.1088, 46.4185) centre (83.1088, 46.482) ccw
  arc A895 (83.1088, 46.4185) -> (83.1088, 46.5455) centre (83.1088, 46.482) ccw
  arc A896 (82.504, 47.5398) -> (82.504, 47.5402) centre (82.504, 47.54) ccw
  arc A897 (82.504, 46.4402) -> (82.504, 46.4398) centre (82.504, 46.44) ccw
  arc A898 (82.4992, 46.5455) -> (82.4992, 46.4185) centre (82.4992, 46.482) ccw
  line L1569 (82.504, 47.54) -> (82.504, 46.44)
  line L1570 (82.804, 47.665) -> (82.804, 47.115)
  line L1571 (82.4992, 46.865) -> (83.1088, 46.865)
  line L1572 (82.804, 47.665) -> (82.804, 47.115)
  arc A899 (85.2588, 50.373) -> (85.2592, 50.373) centre (85.259, 50.373) ccw
  arc A900 (83.1088, 47.5615) -> (83.1088, 47.4345) centre (83.1088, 47.498) ccw
  arc A901 (84.1592, 50.373) -> (84.1588, 50.373) centre (84.159, 50.373) ccw
  arc A902 (83.1088, 47.4345) -> (83.1088, 47.5615) centre (83.1088, 47.498) ccw
  line L1573 (82.804, 46.865) -> (82.804, 46.315)
  arc A903 (82.4992, 46.5455) -> (82.4992, 46.4185) centre (82.4992, 46.482) ccw
  arc A904 (85.2805, 50.9778) -> (85.1535, 50.9778) centre (85.217, 50.9778) ccw
  line L1574 (82.804, 46.865) -> (82.804, 46.315)
  arc A905 (84.1588, 50.373) -> (84.1592, 50.373) centre (84.159, 50.373) ccw
  line L1575 (83.1088, 46.482) -> (82.4992, 46.482)
  arc A906 (82.504, 46.4398) -> (82.504, 46.4402) centre (82.504, 46.44) ccw
  arc A907 (83.104, 46.4402) -> (83.104, 46.4398) centre (83.104, 46.44) ccw
  line L1576 (82.4992, 47.115) -> (82.4992, 46.865)
  line L1577 (82.4992, 47.498) -> (83.1088, 47.498)
  line L1578 (83.1088, 47.498) -> (83.1088, 46.482)
  arc A908 (82.4992, 47.5615) -> (82.4992, 47.4345) centre (82.4992, 47.498) ccw
  line L1579 (83.104, 47.54) -> (82.504, 47.54)
  arc A909 (83.1088, 47.5615) -> (83.1088, 47.4345) centre (83.1088, 47.498) ccw
  line L1580 (82.504, 46.44) -> (83.104, 46.44)
  line L1581 (84.159, 50.973) -> (84.159, 50.373)
  line L1582 (85.217, 50.3682) -> (84.201, 50.3682)
  line L1583 (85.259, 50.373) -> (85.259, 50.973)
  line L1584 (83.1088, 46.865) -> (83.1088, 47.115)
  line L1585 (82.804, 46.865) -> (82.804, 46.315)
  arc A910 (83.1088, 46.5455) -> (83.1088, 46.4185) centre (83.1088, 46.482) ccw
  arc A911 (84.1592, 50.973) -> (84.1588, 50.973) centre (84.159, 50.973) ccw
  line L1586 (84.201, 50.3682) -> (84.201, 50.9778)
  arc A912 (82.4992, 46.4185) -> (82.4992, 46.5455) centre (82.4992, 46.482) ccw
  arc A913 (85.2592, 50.973) -> (85.2588, 50.973) centre (85.259, 50.973) ccw
  line L1587 (82.4992, 46.482) -> (82.4992, 47.498)
  line L1588 (83.1088, 47.115) -> (82.4992, 47.115)
  arc A914 (82.4992, 47.5615) -> (82.4992, 47.4345) centre (82.4992, 47.498) ccw
  arc A915 (83.104, 47.5398) -> (83.104, 47.5402) centre (83.104, 47.54) ccw
  arc A916 (82.4992, 47.4345) -> (82.4992, 47.5615) centre (82.4992, 47.498) ccw
  arc A917 (85.1535, 50.3682) -> (85.2805, 50.3682) centre (85.217, 50.3682) ccw
  arc A918 (84.1375, 49.2252) -> (84.2645, 49.2252) centre (84.201, 49.2252) ccw
  arc A919 (85.2805, 50.9778) -> (85.1535, 50.9778) centre (85.217, 50.9778) ccw
  arc A920 (84.1375, 49.8348) -> (84.2645, 49.8348) centre (84.201, 49.8348) ccw
  line L1589 (84.584, 49.8348) -> (84.584, 49.2252)
  line L1590 (84.201, 49.2252) -> (84.201, 49.8348)
  arc A921 (85.2592, 49.23) -> (85.2588, 49.23) centre (85.259, 49.23) ccw
  arc A922 (84.1375, 50.3682) -> (84.2645, 50.3682) centre (84.201, 50.3682) ccw
  line L1591 (84.034, 49.53) -> (84.584, 49.53)
  arc A923 (85.2588, 49.23) -> (85.2592, 49.23) centre (85.259, 49.23) ccw
  line L1592 (84.034, 50.673) -> (84.584, 50.673)